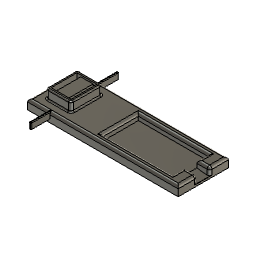
banc de test lineaire GY 521 (Autodesk Fusion 360 design; units mm, degrees)
Autodesk Fusion 360 part; units mm, degrees
sketch "Esquisse1" plane through (0, 0, 0) normal (0, 0, 1) x (1, 0, 0)
  line L0 (0, 0) -> (120, 0)
  line L1 (120, 0) -> (120, 40)
  line L2 (120, 40) -> (0, 40)
  line L3 (0, 40) -> (0, 0)
  dimension "d1" = 120
  dimension "d2" = 40
  constraint horizontal L0
  constraint vertical L1
  constraint horizontal L2
  constraint vertical L3
  constraint coincident L0.start L3.end
  measures "d1" distance of L0.start L0.end
  measures "d2" distance of L0.start L2.end
extrude "Extrusion1" add sketch "Esquisse1" along normal blind 7.5
sketch "Esquisse3" plane through (0, 0, 7.5) normal (0, 0, 1) x (-1, 0, 0)
  line L0 (0, -40) -> (0, 0)
  line L1 (0, 0) -> (-120, 0)
  line L2 (-120, 0) -> (-120, -40)
  line L3 (-120, -40) -> (0, -40)
  line L4 (-110, -5.75) -> (-54, -5.75)
  line L5 (-54, -5.75) -> (-54, -34.25)
  line L6 (-54, -34.25) -> (-110, -34.25)
  line L7 (-110, -34.25) -> (-110, -5.75)
  line L8 (-110, -5.75) -> (-54, -34.25) construction
  line L9 (-54, -5.75) -> (-110, -34.25) construction
  line L10 (-110, -15) -> (-120, -15)
  line L11 (-120, -15) -> (-120, -25)
  line L12 (-120, -25) -> (-110, -25)
  line L13 (-110, -15) -> (-120, -25) construction
  line L14 (-120, -15) -> (-110, -25) construction
  point P0 (-82, -20)
  point P1 (-115, -20)
  dimension "d7" = 56
  dimension "d8" = 28.5
  dimension "d9" = 10
  dimension "d10" = 10
  constraint horizontal L4
  constraint perpendicular L4 L5
  constraint parallel L4 L6
  constraint parallel L5 L7
  constraint coincident L8 P0
  constraint coincident L9 P0
  constraint horizontal L10
  constraint perpendicular L10 L11
  constraint parallel L10 L12
  constraint coincident L13 P1
  constraint coincident L14 P1
  measures "d7" distance of L5.end L6.end
  measures "d8" distance of L4.end L5.end
  measures "d9" distance of L2 L7
  measures "d10" distance of L10.end L11.end
extrude "Extrusion3" cut sketch "Esquisse3" against normal blind 6 contours L2 L7 L10 L11 L12
extrude "Extrusion2" cut sketch "Esquisse3" against normal blind 5 contours L4 L5 L6 L7
sketch "Esquisse4" plane through (0, 0, 7.5) normal (0, 0, 1) x (-1, 0, 0)
  line L0 (-110, -15) -> (-110, -5.75)
  line L1 (-110, -5.75) -> (-54, -5.75)
  line L2 (-54, -5.75) -> (-54, -34.25)
  line L3 (-54, -34.25) -> (-110, -34.25)
  line L4 (-110, -34.25) -> (-110, -25)
  line L5 (-110, -25) -> (-120, -25)
  line L6 (-120, -25) -> (-120, -40)
  line L7 (-120, -40) -> (0, -40)
  line L8 (0, -40) -> (0, 0)
  line L9 (0, 0) -> (-120, 0)
  line L10 (-120, 0) -> (-120, -15)
  line L11 (-120, -15) -> (-110, -15)
  line L12 (-27, -7.5) -> (-7, -7.5)
  line L13 (-7, -7.5) -> (-7, -32.5)
  line L14 (-7, -32.5) -> (-27, -32.5)
  line L15 (-27, -32.5) -> (-27, -7.5)
  line L16 (-27, -7.5) -> (-7, -32.5) construction
  line L17 (-7, -7.5) -> (-27, -32.5) construction
  line L18 (0, 0) -> (-120, 0)
  line L19 (-17, -20) -> (-17, 0) construction
  line L20 (-17, -20) -> (-17, -40) construction
  point P0 (-17, -20)
  dimension "d15" = 20
  dimension "d16" = 25
  dimension "d21" = 7.5
  dimension "d34" = 7
  constraint horizontal L12
  constraint perpendicular L12 L13
  constraint parallel L12 L14
  constraint parallel L13 L15
  constraint coincident L16 P0
  constraint coincident L17 P0
  constraint coincident P0 L19.start
  constraint coincident L9 L19.end
  constraint perpendicular L9 L19
  constraint perpendicular L14 L20
  measures "d15" distance of L13.end L14.end
  measures "d16" distance of L12.end L13.end
  measures "d21" distance of L12 L18
  measures "d34" distance of L8 L13
extrude "Extrusion4" add sketch "Esquisse4" along normal blind 7.5 contours L12 L13 L14 L15
sketch "Esquisse5" plane through (0, 0, 15) normal (0, 0, 1) x (-1, 0, 0)
  line L0 (-27, -32.5) -> (-7, -32.5)
  line L1 (-7, -32.5) -> (-7, -7.5)
  line L2 (-7, -7.5) -> (-27, -7.5)
  line L3 (-27, -7.5) -> (-27, -32.5)
  line L4 (-7, -32.5) -> (-27, -7.5) construction
  line L5 (-27, -32.5) -> (-7, -7.5) construction
  line L6 (-24.925, -9.7) -> (-9.075, -9.7)
  line L7 (-9.075, -9.7) -> (-9.075, -30.3)
  line L8 (-9.075, -30.3) -> (-24.925, -30.3)
  line L9 (-24.925, -30.3) -> (-24.925, -9.7)
  line L10 (-24.925, -9.7) -> (-9.075, -30.3) construction
  line L11 (-9.075, -9.7) -> (-24.925, -30.3) construction
  point P0 (-17, -20)
  dimension "d22" = 15.85
  dimension "d23" = 20.6
  constraint coincident L0.end L1.start
  constraint coincident L2.end L3.start
  constraint coincident L0.start L3.end
  constraint coincident L1.end L2.start
  constraint horizontal L6
  constraint perpendicular L6 L7
  constraint parallel L6 L8
  constraint parallel L7 L9
  constraint coincident L10 P0
  constraint coincident L11 P0
  constraint midpoint L4 P0
  measures "d22" distance of L7.end L8.end
  measures "d23" distance of L6.end L7.end
extrude "Extrusion5" cut sketch "Esquisse5" against normal blind 1.3 contours L6 L7 L8 L9
sketch "Esquisse6" plane through (0, 0, 13.7) normal (0, 0, 1) x (-1, 0, 0)
  line L0 (-24.925, -30.3) -> (-9.075, -30.3)
  line L1 (-9.075, -30.3) -> (-9.075, -9.7)
  line L2 (-9.075, -9.7) -> (-24.925, -9.7)
  line L3 (-24.925, -9.7) -> (-24.925, -30.3)
  line L4 (-9.075, -30.3) -> (-12.075, -30.3)
  line L5 (-12.075, -30.3) -> (-12.075, -9.7)
  line L6 (-12.075, -9.7) -> (-9.075, -9.7)
  line L7 (-9.075, -9.7) -> (-9.075, -30.3)
  line L8 (-24.925, -9.7) -> (-21.925, -9.7)
  line L9 (-21.925, -9.7) -> (-21.925, -30.3)
  line L10 (-21.925, -30.3) -> (-24.925, -30.3)
  line L11 (-24.925, -30.3) -> (-24.925, -9.7)
  dimension "d26" = 3
  dimension "d27" = 3
  constraint horizontal L4
  constraint vertical L5
  constraint horizontal L6
  constraint vertical L7
  constraint coincident L0.end L1.start
  constraint horizontal L8
  constraint vertical L9
  constraint horizontal L10
  constraint vertical L11
  constraint coincident L2.end L3.start
  measures "d26" distance of L0.end L4.end
  measures "d27" distance of L2.end L8.end
extrude "Extrusion6" cut sketch "Esquisse6" against normal blind 3 contours L0 L2 L3 L8 L9 L10 L11 | L0 L1 L2 L4 L5 L6 L7
sketch "Esquisse9" plane through (0, 0, 0) normal (0, -1, 0) x (1, 0, 0)
  line L0 (0, 0) -> (120, 0)
  line L1 (120, 0) -> (120, 7.5)
  line L2 (120, 7.5) -> (0, 7.5)
  line L3 (0, 7.5) -> (0, 0)
  line L4 (17, 0) -> (17, 7.5) construction
  line L5 (17.75, 0) -> (16.25, 0)
  line L6 (16.25, 0) -> (16.25, 7.5)
  line L7 (16.25, 7.5) -> (17.75, 7.5)
  line L8 (17.75, 7.5) -> (17.75, 0)
  line L9 (17.75, 0) -> (16.25, 7.5) construction
  line L10 (16.25, 0) -> (17.75, 7.5) construction
  point P0 (17, 3.75)
  dimension "d35" = 1.5
  constraint coincident L0 L4.start
  constraint coincident L2 L4.end
  constraint perpendicular L2 L4
  constraint horizontal L5
  constraint perpendicular L5 L6
  constraint parallel L5 L7
  constraint parallel L6 L8
  constraint coincident L9 P0
  constraint coincident L10 P0
  constraint midpoint L4 P0
  measures "d35" distance of L6.end L7.end
extrude "Extrusion9" add sketch "Esquisse9" along normal blind 15 contours L0 L2 L5 L6 L7 L8
extrude "Extrusion8" add sketch "Esquisse9" against normal blind 55 contours L0 L2 L5 L6 L7 L8
sketch "Esquisse10" plane through (0, -15, 0) normal (0, -1, 0) x (1, 0, 0)
  line L0 (17.75, 7.5) -> (16.25, 7.5)
  line L1 (16.25, 7.5) -> (16.25, 0)
  line L2 (16.25, 0) -> (17.75, 0)
  line L3 (17.75, 0) -> (17.75, 7.5)
  line L4 (16.25, 0) -> (17.75, 0)
  line L5 (17.75, 0) -> (17.75, 2.6)
  line L6 (17.75, 2.6) -> (16.25, 2.6)
  line L7 (16.25, 2.6) -> (16.25, 0)
  dimension "d40" = 2.6
  constraint horizontal L4
  constraint vertical L5
  constraint horizontal L6
  constraint vertical L7
  constraint coincident L1.end L2.start
  measures "d40" distance of L1.end L6.end
extrude "Extrusion10" cut sketch "Esquisse10" against normal blind 15 contours L1 L2 L3 L4 L5 L6 L7
sketch "Esquisse11" plane through (0, 55, 0) normal (0, 1, 0) x (-1, 0, 0)
  line L0 (-16.25, 7.5) -> (-17.75, 7.5)
  line L1 (-17.75, 7.5) -> (-17.75, 0)
  line L2 (-17.75, 0) -> (-16.25, 0)
  line L3 (-16.25, 0) -> (-16.25, 7.5)
  line L4 (-17.75, 0) -> (-16.25, 0)
  line L5 (-16.25, 0) -> (-16.25, 2.6)
  line L6 (-16.25, 2.6) -> (-17.75, 2.6)
  line L7 (-17.75, 2.6) -> (-17.75, 0)
  dimension "d43" = 2.6
  constraint horizontal L4
  constraint vertical L5
  constraint horizontal L6
  constraint vertical L7
  constraint coincident L1.end L2.start
  measures "d43" distance of L1.end L6.end
extrude "Extrusion11" cut sketch "Esquisse11" against normal blind 15 contours L1 L2 L3 L4 L5 L6 L7
fillet "Congé1" radius 2 7 edges at (82, 34.25, 7.5) (54, 20, 7.5) (82, 5.75, 7.5) (110, 10.375, 7.5) (110, 29.625, 7.5) (115, 25, 7.5) (115, 15, 7.5)
fillet "Congé2" radius 2 11 edges at (68.875, 0, 7.5) (68.875, 40, 7.5) (8.125, 0, 7.5) (0, 20, 7.5) (120, 25, 3.5) (120, 25.5858, 6.9142) (120, 33.5, 7.5) (120, 6.5, 7.5) (120, 14.4142, 6.9142) (120, 15, 3.5) (8.125, 40, 7.5)
fillet "Congé3" radius 1 4 edges at (17, 7.5, 15) (27, 20, 15) (17, 32.5, 15) (7, 20, 15)
fillet "Congé4" radius 2 8 edges at (7, 32.5, 10.75) (7.2929, 32.2071, 14.7071) (7, 7.5, 10.75) (7.2929, 7.7929, 14.7071) (27, 7.5, 10.75) (26.7071, 7.7929, 14.7071) (27, 32.5, 10.75) (26.7071, 32.2071, 14.7071)
fillet "Congé5" radius 1 8 edges at (7.5858, 31.9142, 7.5) (17, 32.5, 7.5) (26.4142, 31.9142, 7.5) (27, 20, 7.5) (26.4142, 8.0858, 7.5) (17, 7.5, 7.5) (7.5858, 8.0858, 7.5) (7, 20, 7.5)
fillet "Congé6" radius 48.5 1 edges at (110, 20, 1.5)
fillet "Congé7" radius 0.5 10 edges at (16.25, -6.5, 7.5) (17.75, -6.5, 7.5) (17, -15, 7.5) (17.75, -15, 5.05) (16.25, -15, 5.05) (16.25, 46.5, 7.5) (17, 55, 7.5) (17.75, 46.5, 7.5) (17.75, 55, 5.05) (16.25, 55, 5.05)
